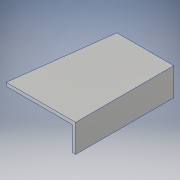
# Autodesk Inventor part: BlockForShieldPlacement
Saved by Autodesk Inventor 2018.3 (Build 223284000, 284)
## iProperties
Created: 2020-02-15
Part Number: BlockForShieldPlacement
Material: Aluminum 6061
Document SubType Name: Modeling
Designer: 22oktynich
Density: 2.7 g/cm^3
Appearance: Aluminum - Flat
Author: 22oktynich
Autodesk Inventor part; units mm, degrees
sketch "Sketch3" plane through (0, 0, 0) normal (0, 0, 1) x (1, 0, 0)
  line L0 (0, 0) -> (0, 76.2)
  line L1 (0, 76.2) -> (-76.2, 76.2)
  line L2 (-76.2, 73.025) -> (-3.175, 73.025)
  line L3 (-3.175, 73.025) -> (-3.175, 0)
  line L4 (-76.2, 73.025) -> (-76.2, 76.2)
  line L5 (-3.175, 0) -> (0, 0)
  dimension "d8" = 76.2
  dimension "d9" = 76.2
  dimension "d10" = 3.175
  constraints: 12 end point, 3 perpendicular, 2 vertical, 1 other
  measures "d8" distance of L0.end L1.end
  measures "d9" distance of L0.start L0.end
  measures "d10" distance between parallel lines of L1 L2
extrude "Extrusion2" add sketch "Sketch3" along normal blind 101.6
sketch "Sketch4" plane through (-76.2, 76.2, 0) normal (0, 1, 0) x (1, 0, 0)
  line L0 (24.13, -11.7529) -> (12.7, -101.6)
  line L1 (0, 0) -> (0, -101.6) projected
  line L2 (24.13, -11.7529) -> (76.2, -11.7529)
  line L3 (76.2, 0) -> (0, 0) projected
  line L4 (76.2, 0) -> (0, 0)
  line L5 (76.2, 0) -> (76.2, -11.7529)
  line L6 (12.7, -101.6) -> (0, -101.6)
  line L7 (0, 0) -> (0, -101.6)
  line L8 (76.2, 0) -> (76.2, -101.6) projected
  dimension "d16" = 7.25
  dimension "d17" = 63.5
  dimension "d18" = 52.07
  constraints: 12 end point, 2 horizontal, 1 perpendicular, 1 vertical
  measures "d16" angle of L1 L0
  measures "d17" distance from line of L8 L0.end
  measures "d18" distance from line of L8 L0.start
extrude "Extrusion3" cut sketch "Sketch4" against normal blind 76.2
ref_plane "Work Plane4" through (-3.175, 0, 101.6) normal (0, -0.7071, 0.7071) x (1, 0, 0)
ref_plane "Work Plane6" through (-63.5, 65.8978, 101.6) normal (0.1262, 0, -0.992) x (0, -1, 0)
sketch "Sketch6" plane through (0, 0, 101.6) normal (1, 0, 0) x (0, 0, -1)
  line L0 (0, 0) -> (0, 76.2) projected
  line L1 (0, 50.8) -> (89.8471, 50.8)
  line L2 (89.8471, 0) -> (0, 0) projected
  line L3 (89.8471, 50.8) -> (89.8471, 0)
  line L4 (89.8471, 0) -> (0, 0)
  line L5 (0, 0) -> (0, 50.8)
  point P0 (101.6, 0)
  dimension "d34" = 50.8
  constraints: 8 end point, 2 perpendicular, 1 collinear, 1 horizontal, 1 point on line
  measures "d34" distance between parallel lines of L2 L1
extrude "Extrusion5" cut sketch "Sketch6" against normal blind 25.4
ref_plane "Work Plane7" through (0, 50.8, 11.7529) normal (0, -0.7071, -0.7071) x (-1, 0, 0)
body "Solid2"
